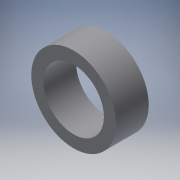
# Autodesk Inventor part: SR-T-08
Saved by Autodesk Inventor 2019.4 (Build 234330000, 330)
## iProperties
Created: 2019-06-15
Part Number: SR-T-08
Material: 一般
Document SubType Name: Modeling
Designer: Koki Shinjo
Mass: 0.0509126 g
Surface Area: 1.39524 cm^2
Volume: 0.0509126 cm^3
Density: 1 g/cm^3
Appearance: 既定
Author: Koki Shinjo
Autodesk Inventor part; units mm, degrees
ref_plane "YZ Plane" through (0, 0, 0) normal (1, 0, 0) x (0, 1, 0)
sketch "スケッチ1" plane through (0, 0, 0) normal (0, 0, 1) x (1, 0, 0)
  line L0 (-0.5912, 0.2511) -> (-0.528, 0.2467) construction
  arc A0 (-0.5749, -0.424) -> (-0.5912, 0.2511) centre (3, 0) ccw construction
  line L1 (-0.528, 0.2467) -> (-0.5749, -0.424) construction
  line L2 (1.8544, -0.9959) -> (0.8585, 0.1498) construction
  arc A1 (1.8544, -0.9959) -> (2.0041, 1.1456) centre (3, 0) ccw construction
  line L3 (0.8585, 0.1498) -> (2.0041, 1.1456) construction
  circle A2 centre (3, 0) radius 3.5
  circle A3 centre (3, 0) radius 2.5
  point P0 (0, 0)
  dimension "d0" = 7
  dimension "d1" = 5
  constraints: 2 centre point, 2 coincident
  measures "d0" diameter of A2
  measures "d1" diameter of A3
ref_plane "作業平面1" through (-0.1209, 6.7653, -3.501) normal (0, 0, 1) x (1, 0, 0)
extrude "押し出し1" add sketch "スケッチ1" against normal up to surface (3.501 mm away)
ref_plane "作業平面2" through (3, 0, -2.701) normal (0, 0, -1) x (-0.0697565, -0.9975641, 0)
sketch "スケッチ2" plane through (3, 0, -2.701) normal (0, 0, -1) x (-0.0697565, -0.9975641, 0)
  circle A0 centre (0, 0) radius 3.5 projected
  circle A1 centre (0, 0) radius 4
  point P0 (0.2093, 2.9927)
  dimension "d4" = 8
  constraints: 1 centre point, 1 coincident
  measures "d4" diameter of A1
extrude "押し出し2" add sketch "スケッチ2" along normal up to surface (0.8 mm away)
move faces "移動1" translate (0, 0, 0.8) faces at (6.1328, 0.2792, -3.501) (3.2756, -3.8019, -3.501)
